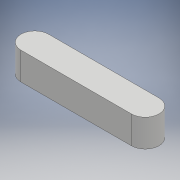
# Autodesk Inventor part: キー
Saved by Autodesk Inventor 2017 (Build 210142000, 142)
## iProperties
Part Number: キー
Material: 一般
Document SubType Name: Modeling
Designer: highs
Density: 1 g/cm^3
Appearance: 既定
Author: highs
Autodesk Inventor part; units mm, degrees
ref_plane "YZ Plane" through (0, 0, 0) normal (1, 0, 0) x (0, 1, 0)
ref_plane "XZ Plane" through (0, 0, 0) normal (0, 1, 0) x (-1, 0, 0)
ref_plane "XY Plane" through (0, 0, 0) normal (0, 0, 1) x (1, 0, 0)
sketch "スケッチ1" plane through (0, 0, 0) normal (0, 0, 1) x (1, 0, 0)
  line L0 (0, 0) -> (-16, 0) construction
  line L1 (0, 2) -> (-16, 2)
  line L2 (-16, -2) -> (0, -2)
  arc A0 (0, -2) -> (0, 2) centre (0, 0) ccw
  arc A1 (-16, 2) -> (-16, -2) centre (-16, 0) ccw
  point P0 (-8, 0)
  dimension "d0" = 4
  dimension "d1" = 16
  constraints: 8 end point, 4 point on circle, 4 tangent, 2 centre point, 1 horizontal, 1 midpoint, 1 parallel
  measures "d0" distance between parallel lines of L1 L2
  measures "d1" distance of L0.start L0.end
extrude "押し出し1" add sketch "スケッチ1" along normal blind 4
